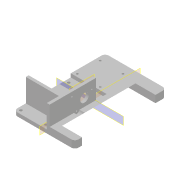
# Autodesk Inventor part: TIRFImager_base_xyz_v0
Saved by Autodesk Inventor 2022 (Build 260153000, 153)
## iProperties
Created: 2022-05-21
Part Number: TIRFImager_base_xyz_v0
Material: Generisch
Document SubType Name: Modeling
Designer: diederichbenedict
Density: 1 g/cm^3
Appearance: Vorgabe
Author: diederichbenedict
Autodesk Inventor part; units mm, degrees
ref_plane "Arbeitsebene4" through (-41.55, 10, -74.35) normal (0, -1, 0) x (1, 0, 0)
sketch "Skizze1" plane through (0, 0, 0) normal (0, 1, 0) x (-1, 0, 0)
  line L0 (-37.75, -63.9) -> (37.75, -63.9)
  line L1 (42.75, -58.9) -> (42.75, 58.9)
  line L2 (37.75, 63.9) -> (-37.75, 63.9)
  line L3 (-42.75, 58.9) -> (-42.75, -58.9)
  line L4 (-42.75, -63.9) -> (42.75, 63.9) construction
  line L5 (42.75, -63.9) -> (-42.75, 63.9) construction
  arc A0 (42.75, 58.9) -> (37.75, 63.9) centre (37.75, 58.9) ccw
  arc A1 (-37.75, 63.9) -> (-42.75, 58.9) centre (-37.75, 58.9) ccw
  arc A2 (-42.75, -58.9) -> (-37.75, -63.9) centre (-37.75, -58.9) ccw
  arc A3 (37.75, -63.9) -> (42.75, -58.9) centre (37.75, -58.9) ccw
  point P0 (0, 0)
  dimension "d0" = 85.5
  dimension "d1" = 127.8
  dimension "d2" = 5
  constraints: 12 end point, 8 point on circle, 8 point on line, 8 tangent, 4 centre point, 3 equal radius, 2 midpoint, 2 parallel, 1 horizontal, 1 perpendicular
  measures "d0" distance of L5.end L4.end
  measures "d1" distance of L4.end L5.start
  measures "d2" radius of A0
extrude "Extrusion1" add sketch "Skizze1" along normal up to surface (10 mm away)
ref_plane "Arbeitsebene1" through (37.75, 0, 0) normal (0, 0, -1) x (-1, 0, 0)
ref_plane "Arbeitsebene2" through (0, 0, 58.9) normal (1, 0, 0) x (0, 0, -1)
sketch "Skizze10" plane through (0, 0, 0) normal (0, -1, 0) x (1, 0, 0)
  circle A0 centre (-37.55, -51.85) radius 1.75 projected
  circle A1 centre (-37.55, -19.85) radius 1.75 projected
  circle A2 centre (-5.55, -51.85) radius 1.75 projected
  circle A3 centre (-5.55, -19.85) radius 1.75 projected
  circle A4 centre (-37.55, -51.85) radius 1.4
  point P0 (0, 0)
  dimension "d37" = 2.8
  constraints: 1 centre point, 1 coincident
  measures "d37" diameter of A4
hole "Bohrung2" at (-37.55, 0, -51.85) at (-37.55, 0, -19.85) at (-5.55, 0, -19.85) at (-5.55, 0, -51.85) direction (0, 1, 0) diameter 2.8 end through all counterbore diameter 6.5 counterbore depth 3.5
sketch "Skizze11" plane through (-37.75, 10, -63.9) normal (0, 1, 0) x (1, 0, 0)
  line L0 (-6.8, -63.05) -> (41.2, -63.05) projected
  line L1 (-6.8, -95.05) -> (41.2, -95.05) projected
  line L2 (-3.8, -48.05) -> (36.2, -48.05) projected
  line L3 (-5, -5) -> (-5, -122.8) projected
  line L4 (0, -127.8) -> (75.5, -127.8) projected
  line L5 (-5, -48.05) -> (45.2, -48.05)
  line L6 (45.2, -48.05) -> (45.2, -127.8)
  line L7 (45.2, -127.8) -> (-5, -127.8)
  line L8 (-5, -127.8) -> (-5, -48.05)
  line L9 (45.2, -108.7984) -> (45.2, -60.5539)
  line L10 (80.5, -82.3) -> (60.5, -82.3) construction
  line L11 (60.5, -82.3) -> (60.5, -82.05) construction
  line L12 (60.5, -82.05) -> (60.5, -81.8) construction
  line L13 (60.5, -81.8) -> (60.5, -81.55) construction
  line L14 (60.5, -81.55) -> (60.5, -81.3) construction
  line L15 (60.5, -81.3) -> (60.5, -81.05) construction
  line L16 (60.5, -81.05) -> (60.5, -80.8) construction
  line L17 (60.5, -80.8) -> (60.5, -80.55) construction
  line L18 (60.5, -80.55) -> (60.5, -80.3) construction
  line L19 (60.5, -80.3) -> (60.5, -80.05) construction
  line L20 (60.5, -80.05) -> (60.5, -79.8) construction
  line L21 (60.5, -79.8) -> (60.5, -79.55) construction
  line L22 (60.5, -79.55) -> (60.5, -79.3) construction
  line L23 (60.5, -79.3) -> (60.5, -79.05) construction
  line L24 (60.5, -79.05) -> (60.5, -78.8) construction
  line L25 (60.5, -78.8) -> (60.5, -78.55) construction
  line L26 (60.5, -78.55) -> (60.5, -78.3) construction
  line L27 (60.5, -78.3) -> (60.5, -78.05) construction
  line L28 (60.5, -78.05) -> (60.5, -77.8) construction
  line L29 (60.5, -77.8) -> (60.5, -77.55) construction
  line L30 (60.5, -77.55) -> (60.5, -77.3) construction
  line L31 (60.5, -77.3) -> (80.5, -77.3) construction
  line L32 (80.5, -77.3) -> (80.5, -41.8) construction
  line L33 (80.5, -41.8) -> (54.7, -41.8) construction
  line L34 (54.7, -41.8) -> (54.7, -117.8) construction
  line L35 (54.7, -117.8) -> (80.5, -117.8) construction
  line L36 (80.5, -117.8) -> (80.5, -82.3) construction
  point P0 (37.75, -63.9)
  dimension "d45" = 0
  constraints: 10 end point, 2 parallel, 2 point on line, 1 horizontal, 1 perpendicular, 1 vertical, 2 other
  measures "d45" distance between parallel lines of L6 L9
ref_plane "Arbeitsebene5" through (-44.55, 5, -0.85) normal (0, -1, 0) x (1, 0, 0)
extrude "Extrusion9" cut sketch "Skizze11" against normal up to surface (5 mm away)
sketch "Skizze12" plane through (0, 0, 0) normal (0, -1, 0) x (1, 0, 0)
  circle A0 centre (-39.55, 15.15) radius 1.4 projected
  circle A1 centre (-11.55, 15.15) radius 1.4 projected
  line L0 (-11.55, 15.15) -> (-39.55, 15.15) construction
  line L1 (-11.55, 16.75) -> (-39.55, 16.75)
  line L2 (-39.55, 13.55) -> (-11.55, 13.55)
  arc A2 (-11.55, 13.55) -> (-11.55, 16.75) centre (-11.55, 15.15) ccw
  arc A3 (-39.55, 16.75) -> (-39.55, 13.55) centre (-39.55, 15.15) ccw
  point P0 (0, 0)
  point P1 (-25.55, 15.15)
  dimension "d48" = 3.2
  constraints: 8 end point, 4 point on circle, 4 tangent, 2 centre point, 1 horizontal, 1 midpoint, 1 parallel
  measures "d48" diameter of A3
extrude "Extrusion10" cut sketch "Skizze12" against normal blind 10 contours A0 | A1 | A2 L2 A3 L1
sketch "Skizze13" plane through (0, 0, 0) normal (0, -1, 0) x (1, 0, 0)
  line L0 (-44.55, 31.15) -> (3.45, 31.15) projected
  line L1 (-11.55, 13.55) -> (-39.55, 13.55) projected
  arc A0 (-39.55, 16.75) -> (-39.55, 13.55) centre (-39.55, 15.15) ccw projected
  line L2 (-39.55, 16.75) -> (-11.55, 16.75) projected
  arc A1 (-11.55, 13.55) -> (-11.55, 16.75) centre (-11.55, 15.15) ccw projected
  arc A2 (-42.75, -58.9) -> (-37.75, -63.9) centre (-37.75, -58.9) ccw projected
  line L3 (37.75, -63.9) -> (-37.75, -63.9) projected
  arc A3 (37.75, -63.9) -> (42.75, -58.9) centre (37.75, -58.9) ccw projected
  line L4 (42.75, 58.9) -> (42.75, -58.9) projected
  arc A4 (42.75, 58.9) -> (37.75, 63.9) centre (37.75, 58.9) ccw projected
  line L5 (-37.75, 63.9) -> (37.75, 63.9) projected
  arc A5 (-37.75, 63.9) -> (-42.75, 58.9) centre (-37.75, 58.9) ccw projected
  line L6 (-42.75, -58.9) -> (-42.75, 58.9) projected
  line L7 (-11.55, 18.4) -> (-39.55, 18.4)
  arc A6 (-39.55, 18.4) -> (-39.55, 11.9) centre (-39.55, 15.15) ccw
  line L8 (-39.55, 11.9) -> (-11.55, 11.9)
  arc A7 (-11.55, 11.9) -> (-11.55, 18.4) centre (-11.55, 15.15) ccw
  point P0 (0, 0)
  dimension "d51" = 6.5
  constraints: 4 end point, 4 point on circle, 2 centre point, 3 other
  measures "d51" distance between parallel lines of L7 L8
extrude "Extrusion11" cut sketch "Skizze13" against normal blind 3 contours L1 A0 L2 A1 | A6 L6 | L6 A6 L7 A7 L8
ref_plane "Arbeitsebene6" through (3.45, 21, 15.15) normal (1, 0, 0) x (0, 0, -1)
sketch "Skizze14" plane through (3.45, 21, 15.15) normal (1, 0, 0) x (0, 0, -1)
  line L0 (16, 16) -> (14, 16) projected
  line L1 (16, -16) -> (16, 16) projected
  line L2 (-16, 16) -> (-16, -16) projected
  circle A0 centre (-17.5, 10) radius 1 construction
  circle A1 centre (-11, -10.5) radius 1 construction
  line L3 (9.4, -16) -> (6.6, -16) projected
  circle A2 centre (10.5, 5) radius 1 construction
  circle A3 centre (0, 0) radius 6 projected
  line L4 (-48.75, -21) -> (-48.75, -11) projected
  line L5 (16, 16) -> (-48.75, 16)
  line L6 (-48.75, 16) -> (-48.75, -16)
  line L7 (-48.75, -16) -> (16, -16)
  line L8 (16, -16) -> (16, 16)
  circle A4 centre (-17.5, 10) radius 0.9
  circle A5 centre (10.5, 5) radius 0.85
  circle A6 centre (-11, -10.5) radius 0.85
  point P0 (15.15, -21)
  point P1 (9.4, -16)
  point P2 (16, -16)
  point P3 (14, 16)
  point P4 (-48.75, -11)
  point P5 (6.6, -16)
  dimension "d56" = 1.8
  dimension "d57" = 1.7
  dimension "d58" = 1.7
  constraints: 8 end point, 3 centre point, 3 coincident, 2 parallel, 1 horizontal, 1 midpoint, 1 perpendicular
  measures "d56" diameter of A4
  measures "d57" diameter of A5
  measures "d58" diameter of A6
ref_plane "Arbeitsebene7" through (7.45, -0.1921, -3.518) normal (-1, 0, 0) x (0, -0.417504, 0.9086751)
extrude "Extrusion12" add sketch "Skizze14" along normal up to surface (4 mm away)
sketch "Skizze15" plane through (-37.75, 10, -63.9) normal (0, 1, 0) x (1, 0, 0)
  line L0 (-5, -48.05) -> (45.2, -48.05) projected
  line L1 (45.2, -48.05) -> (45.2, -63.05) projected
  line L2 (45.2, -63.05) -> (45.2, -89.3626) projected
  line L3 (45.2, -89.3626) -> (45.2, -90.7374) projected
  line L4 (45.2, -90.7374) -> (45.2, -127.8) projected
  line L5 (45.2, -127.8) -> (75.5, -127.8) projected
  arc A0 (75.5, -127.8) -> (80.5, -122.8) centre (75.5, -122.8) ccw projected
  line L6 (80.5, -122.8) -> (80.5, -5) projected
  arc A1 (80.5, -5) -> (75.5, 0) centre (75.5, -5) ccw projected
  line L7 (75.5, 0) -> (0, 0) projected
  arc A2 (0, 0) -> (-5, -5) centre (0, -5) ccw projected
  line L8 (-5, -5) -> (-5, -48.05) projected
  line L9 (80.5, -117.8) -> (52.5869, -117.8)
  line L10 (52.5869, -117.8) -> (52.5869, -15)
  line L11 (52.5869, -15) -> (80.5, -15)
  line L12 (80.5, -15) -> (80.5, -117.8)
  line L13 (45.7, -42.1725) -> (45.7, -1.05)
  point P0 (37.75, -63.9)
  point P1 (80.5, -15)
  dimension "d59" = 10
  dimension "d60" = 15
  constraints: 10 end point, 2 parallel, 1 horizontal, 1 perpendicular, 1 point on line, 1 vertical, 2 other
  measures "d59" distance between parallel lines of L9 L5
  measures "d60" distance between parallel lines of L7 L11
extrude "Extrusion13" cut sketch "Skizze15" against normal through all contours L6 L9 L10 L11
sketch "Skizze16" plane through (7.45, 10, -0.85) normal (1, 0, 0) x (0, 0, -1)
  circle A0 centre (-27, 0.5) radius 1 projected
  circle A1 centre (-27, 0.5) radius 0.85 projected
  circle A2 centre (-27, 0.5) radius 3.8399
  point P0 (-0.85, -10)
  constraints: 1 centre point, 1 coincident
extrude "Extrusion14" cut sketch "Skizze16" along normal up to surface (7.3869 mm away) contours A0 | A1 | A2
chamfer "Fase1" distance 10 angle 45 1 edges at (14.8369, 0, 2.5)
sketch "Skizze17" plane through (-42.75, 5, -15.85) normal (0, 1, 0) x (1, 0, 0)
  line L0 (46.2, -79.75) -> (46.2, -15) projected
  line L1 (46.2, -15) -> (50.2, -15) projected
  line L2 (50.2, -15) -> (50.2, 0) projected
  line L3 (50.2, 0) -> (0, 0) projected
  line L4 (0, -74.75) -> (0, 0) projected
  arc A0 (0, -74.75) -> (5, -79.75) centre (5, -74.75) ccw projected
  line L5 (46.2, -79.75) -> (5, -79.75) projected
  line L6 (3.2, -29.4) -> (31.2, -29.4) projected
  arc A1 (31.2, -32.6) -> (31.2, -29.4) centre (31.2, -31) ccw projected
  line L7 (31.2, -32.6) -> (3.2, -32.6) projected
  arc A2 (3.2, -29.4) -> (3.2, -32.6) centre (3.2, -31) ccw projected
  line L8 (5, -74.75) -> (40, -74.75)
  line L9 (40, -74.75) -> (40, -7.75)
  line L10 (40, -7.75) -> (5, -7.75)
  line L11 (5, -7.75) -> (5, -74.75)
  point P0 (42.75, -15.85)
  dimension "d68" = 35
  dimension "d69" = 67
  constraints: 8 end point, 2 parallel, 1 horizontal, 1 perpendicular
  measures "d68" distance of L10.end L9.end
  measures "d69" distance of L9.end L8.end
hole "Bohrung3" at (-37.75, 5, -8.1) at (-2.75, 5, -8.1) at (-2.75, 5, 58.9) at (-37.75, 5, 58.9) direction (0, -1, 0) diameter 3.8 end through all
sketch "Skizze18" plane through (3.45, 37, 63.9) normal (0, 1, 0) x (1, 0, 0)
  line L0 (4, 64.75) -> (4, 0) projected
  line L1 (0, 64.75) -> (4, 64.75) projected
  line L2 (0, 64.75) -> (0, 0) projected
  line L3 (0, 0) -> (4, 0) projected
  line L4 (-46.2, 5) -> (-46.2, 79.75) projected
  line L5 (0, 16.8478) -> (-46.2, 16.8478)
  line L6 (-46.2, 16.8478) -> (-46.2, 20.8478)
  line L7 (-46.2, 20.8478) -> (0, 20.8478)
  line L8 (0, 20.8478) -> (0, 16.8478)
  point P0 (-3.45, 63.9)
  point P1 (0, 20.8478)
  point P2 (-46.2, 16.8478)
  dimension "d77" = 4
  constraints: 8 end point, 2 parallel, 2 point on line, 1 horizontal, 1 perpendicular
  measures "d77" distance of L5.end L6.end
extrude "Extrusion15" add sketch "Skizze18" against normal up to surface (32 mm away) contours L2 L5 L4 L7
